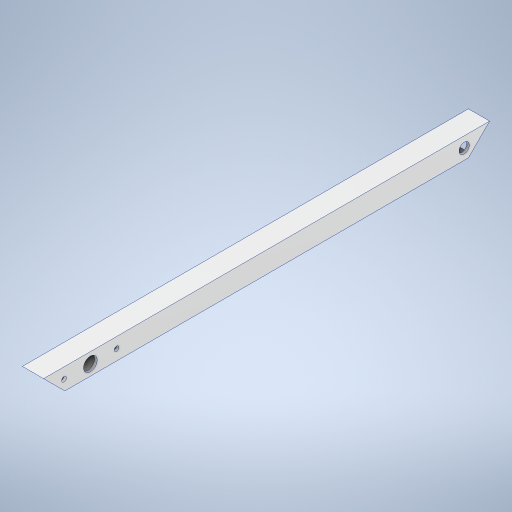
# Autodesk Inventor part: P402
Saved by Autodesk Inventor 2023 (Build 270158000, 158)
## iProperties
Created: 2022-08-29
Part Number: P402
Material: Aluminum 6061
Document SubType Name: Modeling
Designer: D.C. Eksteen
Density: 2.7 g/cm^3
Appearance: Aluminum - Flat
Author: D.C. Eksteen
Title: LEFT REAR TOP TUBE
Autodesk Inventor part; units mm, degrees
ref_plane "YZ Plane" through (0, 0, 0) normal (1, 0, 0) x (0, 1, 0)
ref_plane "XZ Plane" through (0, 0, 0) normal (0, 1, 0) x (-1, 0, 0)
ref_plane "XY Plane" through (0, 0, 0) normal (0, 0, 1) x (1, 0, 0)
sketch "Sketch1" plane through (0, 0, 0) normal (0, 0, 1) x (1, 0, 0)
  line L0 (0, 0) -> (25, 0)
  line L1 (25, 0) -> (25, 25)
  line L2 (25, 25) -> (0, 25)
  line L3 (0, 25) -> (0, 0)
  line L4 (3, 22) -> (22, 22)
  line L5 (22, 22) -> (22, 3)
  line L6 (22, 3) -> (3, 3)
  line L7 (3, 3) -> (3, 22)
  dimension "d0" = 25
  dimension "d1" = 25
  dimension "d2" = 3
  constraints: 16 end point, 4 parallel, 2 perpendicular, 1 horizontal, 3 other
  measures "d0" distance of L2.end L1.end
  measures "d1" distance of L1.end L0.end
  measures "d2" distance between parallel lines of L2 L4
extrude "Extrusion1" add sketch "Sketch1" along normal blind 525
sketch "Sketch2" plane through (25, 0, 0) normal (1, 0, 0) x (0, 0, -1)
  line L0 (0, 0) -> (0, 25) projected
  line L1 (0, 25) -> (-525, 25) projected
  line L2 (-525, 0) -> (-525, 25) projected
  line L3 (0, 0) -> (-525, 0) projected
  line L4 (-525, 25) -> (-500, 0)
  line L5 (-525, 25) -> (-489.6447, 25) construction
  line L6 (0, 25) -> (-25, 0)
  line L7 (0, 25) -> (35.3553, 25) construction
  dimension "d5" = 45
  dimension "d6" = 135
  constraints: 8 end point, 2 equal length, 2 horizontal, 2 point on line
  measures "d5" angle of L4 L5
  measures "d6" angle of L6 L7
extrude "Extrusion2" cut sketch "Sketch2" against normal blind 500 contours L3 L6 L0 | L4 L3 L2
sketch "Sketch3" plane through (25, 25, 525) normal (1, 0, 0) x (0, 0, -1)
  line L0 (500, -25) -> (25, -25) projected
  line L1 (525, 0) -> (0, 0) projected
  line L2 (25, -25) -> (0, 0) projected
  point P0 (525, -25)
  point P1 (55, -12.5)
  point P2 (495, -12.5)
  point P3 (262.5, 0)
  point P4 (12.5, -12.5)
  point P5 (12.5, -12.5)
  dimension "d9" = 440
  dimension "d10" = 12.5
  dimension "d50" = 42.5
  constraints: 3 midpoint, 1 horizontal alignment
  measures "d9" distance of point (495, -12.5) point (55, -12.5)
  measures "d10" distance from line of L0 point (495, -12.5)
  measures "d50" distance of point (12.5, -12.5) point (55, -12.5)
hole "Hole1" at (25, 12.5, 30) direction (-1, 0, 0) diameter 12 depth 8 tip angle 118
sketch "Sketch5" plane through (0, 25, 0) normal (-1, 0, 0) x (0, 0, 1)
  circle A0 centre (30, -12.5) radius 6 projected
  point P0 (0, -25)
  point P1 (470, -12.5)
  dimension "d33" = 440
  constraints: 1 coincident
  measures "d33" distance of point (470, -12.5) point (30, -12.5)
hole "Hole3" at (0, 12.5, 30) at (0, 12.5, 470) direction (1, 0, 0) diameter 8 depth 8 tip angle 118
sketch "Sketch6" plane through (0, 25, 0) normal (-1, 0, 0) x (0, 0, 1)
  circle A0 centre (470, -12.5) radius 4 projected
  point P0 (0, -25)
  constraints: 1 coincident
hole "Hole4" at (0, 12.5, 470) direction (1, 0, 0) diameter 16 end through all
sketch "Sketch7" plane through (0, 25, 0) normal (-1, 0, 0) x (0, 0, 1)
  circle A0 centre (470, -12.5) radius 8 projected
  circle A1 centre (30, -12.5) radius 4 projected
  line L0 (0, 0) -> (25, -25) projected
  line L1 (25, -25) -> (500, -25) projected
  line L2 (500, -25) -> (525, 0) projected
  line L3 (0, 0) -> (525, 0) projected
  circle A2 centre (470, -12.5) radius 31
  line L4 (439, -12.5) -> (501, -12.5)
  point P0 (0, -25)
  dimension "d41" = 62
  constraints: 4 coincident, 2 end point, 2 point on circle, 1 centre point, 1 horizontal, 1 midpoint
  measures "d41" diameter of A2
hole "Hole5" at (0, 12.5, 439) at (0, 12.5, 501) direction (1, 0, 0) diameter 5.5 end through all clearance for "Flat Head Machine Screw" size "M5" standard "Ansi Metric M Profile"
body "Solid1"
